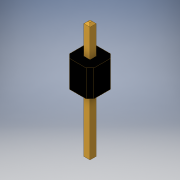
# Autodesk Inventor part: Single Short Male Header
Saved by Autodesk Inventor 2016 (Build 200138000, 138)
## iProperties
Created: 2015-11-30
Part Number: Single Short Male Header
Material: Generic
Document SubType Name: Modeling
Designer: Spooner
Density: 1 g/cm^3
Appearance: Brass - Satin
Author: Spooner
Autodesk Inventor part; units mm, degrees
ref_plane "YZ Plane" through (0, 0, 0) normal (1, 0, 0) x (0, 1, 0)
ref_plane "XZ Plane" through (0, 0, 0) normal (0, 1, 0) x (-1, 0, 0)
ref_plane "XY Plane" through (0, 0, 0) normal (0, 0, 1) x (1, 0, 0)
sketch "Sketch1" plane through (0, 0, 0) normal (0, 1, 0) x (-1, 0, 0)
  line L0 (-1.1938, 1.1938) -> (1.1938, 1.1938)
  line L1 (1.1938, 1.1938) -> (1.1938, -1.1938)
  line L2 (1.1938, -1.1938) -> (-1.1938, -1.1938)
  line L3 (-1.1938, -1.1938) -> (-1.1938, 1.1938)
  line L4 (-1.1938, 1.1938) -> (1.1938, -1.1938) construction
  line L5 (1.1938, 1.1938) -> (-1.1938, -1.1938) construction
  point P0 (0, 0)
  dimension "d0" = 2.3876
  constraints: 12 end point, 2 midpoint, 2 parallel, 2 perpendicular, 1 horizontal
  measures "d0" distance of L0.end L1.end
extrude "Extrusion1" add sketch "Sketch1" along normal blind 2.6035
chamfer "Chamfer1" distance 0.381 angle 45 4 edges at (1.1938, 1.3017, 1.1938) (-1.1938, 1.3017, 1.1938) (1.1938, 1.3017, -1.1938) (-1.1938, 1.3017, -1.1938)
sketch "Sketch2" plane through (0, 2.6035, 0) normal (0, 1, 0) x (1, 0, 0)
  line L0 (0.2984, 0.2984) -> (-0.2984, 0.2984)
  line L1 (-0.2984, 0.2984) -> (-0.2984, -0.2984)
  line L2 (-0.2984, -0.2984) -> (0.2984, -0.2984)
  line L3 (0.2984, -0.2984) -> (0.2984, 0.2984)
  line L4 (0.2984, 0.2984) -> (-0.2984, -0.2984) construction
  line L5 (-0.2984, 0.2984) -> (0.2984, -0.2984) construction
  point P0 (0, 0)
  dimension "d6" = 0.5969
  constraints: 12 end point, 2 midpoint, 2 parallel, 2 perpendicular, 1 horizontal
  measures "d6" distance of L0.end L1.end
extrude "Extrusion2" add sketch "Sketch2" along normal blind 2.921 and the other way blind 8.636
chamfer "Chamfer2" distance 0.1905 angle 45 8 edges at (0.2984, 5.5245, 0) (0, 5.5245, -0.2984) (-0.2984, 5.5245, 0) (0, 5.5245, 0.2984) (0, -6.0325, -0.2984) (0.2984, -6.0325, 0) (0, -6.0325, 0.2984) (-0.2984, -6.0325, 0)
body "Solid1"
